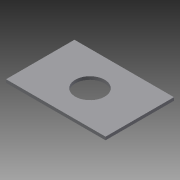
# Autodesk Inventor part: zMotorMount
Saved by Autodesk Inventor 2013 (Build 170138000, 138)
## iProperties
Created: 2012-12-03
Part Number: zMotorMount
Material: Generic
Document SubType Name: Modeling
Designer: istvan.burbank
Density: 1 g/cm^3
Mass: 19.3135 g
Surface Area: 133.007 cm^2
Volume: 19.3135 cm^3
Author: istvan.burbank
Autodesk Inventor part; units mm, degrees
ref_plane "YZ Plane" through (0, 0, 0) normal (1, 0, 0) x (0, 1, 0)
ref_plane "XZ Plane" through (0, 0, 0) normal (0, 1, 0) x (-1, 0, 0)
ref_plane "XY Plane" through (0, 0, 0) normal (0, 0, 1) x (1, 0, 0)
sketch "Sketch1" plane through (0, 0, 0) normal (0, 1, 0) x (-1, 0, 0)
  line L0 (0, 0) -> (101.6, 0)
  line L1 (101.6, 0) -> (101.6, 69.85)
  line L2 (101.6, 69.85) -> (0, 69.85)
  line L3 (0, 69.85) -> (0, 0)
  dimension "d6" = 101.6
  dimension "d7" = 69.85
  constraints: 8 end point, 2 parallel, 1 coincident, 1 horizontal, 1 perpendicular
  measures "d6" distance of L2.end L1.end
  measures "d7" distance of L1.end L0.end
extrude "Extrusion1" add sketch "Sketch1" along normal blind 3.175
sketch "Sketch2" plane through (0, 0, 0) normal (0, -1, 0) x (1, 0, 0)
  line L0 (0, 0) -> (-101.6, 0) projected
  line L1 (0, 69.85) -> (0, 0) projected
  line L2 (-101.6, 69.85) -> (0, 69.85) projected
  line L3 (-101.6, 0) -> (-101.6, 69.85) projected
  circle A0 centre (-50.8, 34.925) radius 15
  dimension "d8" = 30
  dimension "d9" = 50.8
  dimension "d10" = 50.8
  dimension "d11" = 34.925
  dimension "d12" = 34.925
  constraints: 1 centre point
  measures "d8" diameter of A0
  measures "d9" distance from line of L3 A0.centre
  measures "d10" distance from line of L1 A0.centre
  measures "d11" distance from line of L2 A0.centre
  measures "d12" distance from line of L0 A0.centre
extrude "Extrusion2" cut sketch "Sketch2" against normal through all contours A0
equation "\"d9\" = d10"
equation "\"d11\" = d12"
body "Solid1"
